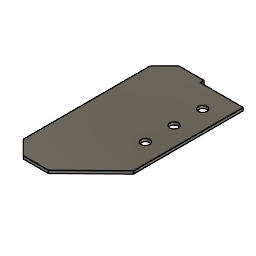
GPL H350 to 250G25_ (Autodesk Fusion 360 design; units mm, degrees)
Autodesk Fusion 360 part; units mm, degrees
sketch "スケッチ1" plane through (0, 0, 0) normal (0, 0, 1) x (1, 0, 0)
  line L0 (-3.5, 163) -> (-86.5, 163)
  line L1 (-86.5, 163) -> (-86.5, -163)
  line L2 (-86.5, -163) -> (-3.5, -163)
  line L3 (86.5, -75) -> (86.5, 155)
  line L4 (82.2546, 155) -> (-86.5, -163) construction
  line L5 (-86.5, 163) -> (55.7541, -105.0627) construction
  line L6 (-3.5, 163) -> (-3.5, 155)
  line L7 (-3.5, 155) -> (86.5, 155)
  line L8 (-86.5, -163) -> (-3.5, -163) construction
  line L9 (86.5, -75) -> (-3.5, -163)
  dimension "d2" = 326
  dimension "d5" = 83
  constraint horizontal L0
  constraint perpendicular L0 L1
  constraint parallel L0 L2
  constraint parallel L1 L3
  constraint coincident L4 origin
  constraint coincident L5 origin
  constraint vertical L6
  constraint horizontal L7
  constraint coincident L7 L4.start
  constraint perpendicular L1 L8
  constraint coincident L9 L5.end
  measures "d2" distance of L0.end L1.end
  measures "d5" distance of L1.end L2.end
extrude "押し出し1" add sketch "スケッチ1" along normal blind 6
chamfer "面取り1" distance 30 angle 45 2 edges at (-86.5, -163, 3) (-86.5, 163, 3)
sketch "スケッチ2" plane through (0, 0, 6) normal (0, 0, 1) x (-1, 0, 0)
  line L0 (56.5, -163) -> (86.5, -133)
  line L1 (86.5, -133) -> (86.5, 133)
  line L2 (86.5, 133) -> (56.5, 163)
  line L3 (56.5, 163) -> (3.5, 163)
  line L4 (3.5, 163) -> (-86.5, 75)
  line L5 (-86.5, 75) -> (-86.5, -155)
  line L6 (-86.5, -155) -> (3.5, -155)
  line L7 (3.5, -155) -> (3.5, -163)
  line L8 (3.5, -163) -> (56.5, -163)
  line L9 (-86.5, -155) -> (-46.5, -155) construction
  line L10 (-46.5, -155) -> (-46.5, -110) construction
  line L11 (-46.5, -110) -> (-86.5, -110) construction
  line L12 (-86.5, -110) -> (-86.5, -155) construction
  line L13 (-46.5, -110) -> (-46.5, -50) construction
  line L14 (-46.5, -50) -> (-46.5, 10) construction
  point P0 (-46.5, -110)
  point P1 (-46.5, -50)
  point P2 (-46.5, 10)
  dimension "d10" = 40
  dimension "d11" = 45
  dimension "d12" = 60
  dimension "d13" = 60
  constraint horizontal L9
  constraint vertical L10
  constraint horizontal L11
  constraint vertical L12
  constraint coincident L5.end L6.start
  constraint perpendicular L11 L13
  constraint parallel L13 L14
  constraint coincident P0 L10.end
  constraint coincident P1 L13.end
  constraint coincident P2 L14.end
  measures "d10" distance of L5.end L9.end
  measures "d11" distance of L5.end L11.end
  measures "d12" distance of P0 P1
  measures "d13" distance of P1 P2
hole "穴1" at (46.5, 110, 6) at (46.5, 50, 6) at (46.5, -10, 6) direction (0, 0, -1) diameter 18 end through all
equation "d5 = 30 mm + 53 mm"
